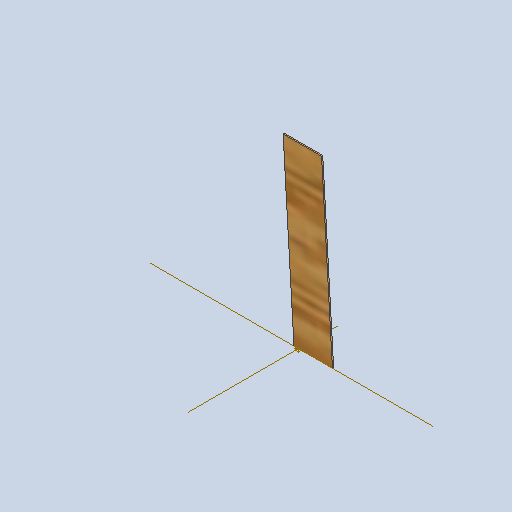
# Autodesk Inventor part: sponson_bottom_indent
Saved by Autodesk Inventor 2022 (Build 260153070, 153G)
## iProperties
Created: 2021-05-05
Part Number: sponson_bottom_indent
Material: Plywood, Sheathing, Epoxy Protected
Document SubType Name: Modeling
Designer: kardo
Density: 0.552 g/cm^3
Appearance: Plywood - New
Mass: 1.47592 g
Surface Area: 69.3138 cm^2
Volume: 2.67376 cm^3
Author: kardo
Autodesk Inventor part; units mm, degrees
ref_plane "YZ Plane" through (0, 0, 0) normal (1, 0, 0) x (0, 1, 0)
ref_plane "XZ Plane" through (0, 0, 0) normal (0, 1, 0) x (-1, 0, 0)
ref_plane "XY Plane" through (0, 0, 0) normal (0, 0, 1) x (1, 0, 0)
derived "frame_outline.ipt"
sketch "joints_sponson_bottom" plane through (81, 0, 0) normal (1, 0, 0) x (0, 1, 0)
  line L0 (0, 0) -> (130.35, 9.115)
  line L1 (0, 4.352) -> (-363, 13.6)
  line L2 (133.5641, -36.8495) -> (121.9065, 129.8631) construction
  line L3 (130.1045, 12.6264) -> (0, 5.1533) construction
  line L4 (130.1603, 11.8283) -> (0, 4.352) construction
  line L5 (0, 5.1533) -> (0, 4.352)
  line L6 (0, 4.352) -> (0, 0)
  line L7 (130.1603, 11.8283) -> (130.35, 9.115)
  line L8 (130.1045, 12.6264) -> (130.1603, 11.8283)
  line L9 (94.8, 86.9585) -> (94.8, -19.4928) construction
  point P0 (94.8, 10.5986)
  point P1 (0, 5.1533)
sketch "bh_main" plane through (0, 0, 0) normal (0, 1, 0) x (-1, 0, 0)
  line L0 (-81, 19.8753) -> (-133.5, 0) construction
  line L1 (-156, 31.008) -> (-133.5, 0) construction
  line L2 (-133.5, 0) -> (-104.625, 0) construction
  line L3 (-81, 4.352) -> (-81, 26.5308) construction
  line L4 (-81, 26.5308) -> (-30, 26.5308) construction
  line L5 (-30, 26.5308) -> (-30, 17.8644) construction
  line L6 (-30, 17.8644) -> (0, 17.8644) construction
  line L7 (-104.625, 0) -> (-81, 0) construction
  line L8 (-81, 4.352) -> (-81, 0) construction
  line L9 (-55, 55.974) -> (0, 55.974) construction
  line L10 (0, 55.174) -> (0, 18.6644)
  line L11 (0, -19.4928) -> (0, 86.9585) construction
  line L12 (0, 55.174) -> (-55, 55.174)
  line L13 (-154.827, 30.7537) -> (-133.0921, 0.8)
  line L14 (-133.0921, 0.8) -> (-81, 0.8)
  line L15 (0, 18.6644) -> (-28, 18.6644)
  line L16 (-28, 18.6644) -> (-28, 27.3308)
  line L17 (-28, 27.3308) -> (-81, 27.3308)
  line L18 (-81, 27.3308) -> (-81, 0.8)
  line L19 (-81, 5.1533) -> (-107.046, 5.1533)
  line L20 (-107.046, 5.1533) -> (-107.046, 0.8)
  spline S0 degree 4 poles (-156, 31.008) (-141.197, 39.4592) (-115.7093, 49.7229) (-91.1756, 54.0594) (-64.7341, 55.974) (-55, 55.974) knots 0 0 0 0 0 0.628223 1 1 1 1 1 construction
  spline S1 degree 3 poles (-55, 55.174) (-57.8721, 55.174) (-62.9171, 55.0523) (-68.6715, 54.7173) (-72.9721, 54.3919) (-75.8302, 54.1391) (-79.3894, 53.7801) (-82.2253, 53.4591) (-85.7552, 53.0157) (-88.5673, 52.6269) (-92.7689, 51.9904) (-96.9501, 51.2808) (-102.5023, 50.1987) (-106.6538, 49.2786) (-110.7984, 48.2651) (-113.5582, 47.5419) (-117.0041, 46.5761) (-119.7575, 45.7532) (-123.1946, 44.6603) (-125.9399, 43.734) (-129.3642, 42.5097) (-132.0971, 41.4769) (-135.5019, 40.1186) (-138.2157, 38.9779) (-142.2664, 37.1856) (-147.6278, 34.6514) (-152.2348, 32.2151) (-154.827, 30.7537) knots 0.008263 0.008263 0.008263 0.008263 0.090908 0.152892 0.173553 0.214875 0.235536 0.276859 0.29752 0.338842 0.359503 0.421487 0.462809 0.524793 0.545454 0.586776 0.607438 0.64876 0.669421 0.710743 0.731405 0.772727 0.793388 0.834711 0.855372 0.917355 1 1 1 1
  point P0 (0, 0)
  point P1 (-81, 40.4654)
ref_plane "plane_stringer_outer" through (84, 0, 0) normal (1, 0, 0) x (0, 1, 0)
ref_plane "Work Plane3" through (81, 130.1045, 12.6264) normal (0, -0.0573449, 0.9983544) x (0, -0.9983544, -0.0573449)
sketch "Sketch5" plane through (81, 130.1045, 12.6264) normal (0, -0.0573449, 0.9983544) x (0, -0.9983544, -0.0573449)
  line L0 (0, 0) -> (130.3189, 0) projected
  line L1 (130.3189, 0) -> (130.3189, 26.046) projected
  line L2 (130.3189, 26.046) -> (0, 26.046)
  line L3 (0, 26.046) -> (0, 0) construction
  line L4 (2, 0) -> (2, 26.046)
  point P0 (130.6144, -81)
  dimension "d6" = 2
  constraints: 6 end point, 3 parallel, 2 point on line
  measures "d6" distance between parallel lines of L3 L4
extrude "Extrusion2" add sketch "Sketch5" against normal blind 0.8
equation "\"d6\" = bulkhead_thickness"
equation "\"d4\" = surface_thickness"
equation "\"bulkhead_thickness\" = 2"
equation "\"surface_thickness\" = 0.8"
body "Solid2"
